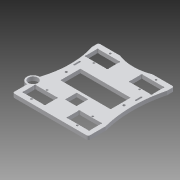
# Autodesk Inventor part: base doble extrusor xl i v1.3
Saved by Autodesk Inventor 2012 SP1 (Build 160190100, 190)
## iProperties
Created: 2015-08-07
Part Number: base doble extrusor xl i v1.3
Material: Default
Document SubType Name: Modeling
Designer: Laser router cnc
Density: 1 g/cm^3
Author: Laser router cnc
Autodesk Inventor part; units mm, degrees
(part 1 of 2)
ref_plane "YZ Plane" through (0, 0, 0) normal (1, 0, 0) x (0, 1, 0)
ref_plane "XZ Plane" through (0, 0, 0) normal (0, 1, 0) x (-1, 0, 0)
ref_plane "XY Plane" through (0, 0, 0) normal (0, 0, 1) x (1, 0, 0)
sketch "Boceto1" plane through (0, 0, 0) normal (0, 0, 1) x (1, 0, 0)
  line L0 (375.8398, -66.6637) -> (375.8398, -81.652)
  line L1 (375.8398, -81.652) -> (361.1315, -81.652)
  line L2 (361.1315, -81.652) -> (361.1315, -66.6637)
  line L3 (361.1315, -66.6637) -> (375.8398, -66.6637)
  line L4 (401.2261, -37.6694) -> (401.2261, -63.2662)
  line L5 (401.2261, -63.2662) -> (336.8198, -63.2662)
  line L6 (336.8198, -63.2662) -> (336.8198, -37.6694)
  line L7 (336.8198, -37.6694) -> (401.2261, -37.6694)
  line L8 (397.7416, -0.2246) -> (397.8694, -0.2311)
  line L9 (397.8694, -0.2311) -> (397.9936, -0.25)
  line L10 (397.9936, -0.25) -> (398.1134, -0.2808)
  line L11 (398.1134, -0.2808) -> (398.2283, -0.3228)
  line L12 (398.2283, -0.3228) -> (398.3376, -0.3754)
  line L13 (398.3376, -0.3754) -> (398.4407, -0.438)
  line L14 (398.4407, -0.438) -> (398.5369, -0.51)
  line L15 (398.5369, -0.51) -> (398.6257, -0.5906)
  line L16 (398.6257, -0.5906) -> (398.7064, -0.6794)
  line L17 (398.7064, -0.6794) -> (398.7784, -0.7756)
  line L18 (398.7784, -0.7756) -> (398.841, -0.8787)
  line L19 (398.841, -0.8787) -> (398.8937, -0.9879)
  line L20 (398.8937, -0.9879) -> (398.9357, -1.1027)
  line L21 (398.9357, -1.1027) -> (398.9665, -1.2225)
  line L22 (398.9665, -1.2225) -> (398.9855, -1.3466)
  line L23 (398.9855, -1.3466) -> (398.9919, -1.4744)
  line L24 (398.9919, -1.4744) -> (398.9855, -1.6022)
  line L25 (398.9855, -1.6022) -> (398.9665, -1.7263)
  line L26 (398.9665, -1.7263) -> (398.9357, -1.8461)
  line L27 (398.9357, -1.8461) -> (398.8937, -1.9609)
  line L28 (398.8937, -1.9609) -> (398.8411, -2.0702)
  line L29 (398.8411, -2.0702) -> (398.7785, -2.1732)
  line L30 (398.7785, -2.1732) -> (398.7065, -2.2695)
  line L31 (398.7065, -2.2695) -> (398.6259, -2.3583)
  line L32 (398.6259, -2.3583) -> (398.5371, -2.4389)
  line L33 (398.5371, -2.4389) -> (398.4409, -2.5109)
  line L34 (398.4409, -2.5109) -> (398.3379, -2.5736)
  line L35 (398.3379, -2.5736) -> (398.2286, -2.6262)
  line L36 (398.2286, -2.6262) -> (398.1138, -2.6683)
  line L37 (398.1138, -2.6683) -> (397.994, -2.6991)
  line L38 (397.994, -2.6991) -> (397.8699, -2.7181)
  line L39 (397.8699, -2.7181) -> (397.7421, -2.7246)
  line L40 (397.7421, -2.7246) -> (397.6143, -2.7182)
  line L41 (397.6143, -2.7182) -> (397.4902, -2.6993)
  line L42 (397.4902, -2.6993) -> (397.3705, -2.6685)
  line L43 (397.3705, -2.6685) -> (397.2556, -2.6265)
  line L44 (397.2556, -2.6265) -> (397.1464, -2.5739)
  line L45 (397.1464, -2.5739) -> (397.0433, -2.5113)
  line L46 (397.0433, -2.5113) -> (396.947, -2.4394)
  line L47 (396.947, -2.4394) -> (396.8583, -2.3587)
  line L48 (396.8583, -2.3587) -> (396.7776, -2.27)
  line L49 (396.7776, -2.27) -> (396.7056, -2.1737)
  line L50 (396.7056, -2.1737) -> (396.643, -2.0707)
  line L51 (396.643, -2.0707) -> (396.5903, -1.9614)
  line L52 (396.5903, -1.9614) -> (396.5482, -1.8466)
  line L53 (396.5482, -1.8466) -> (396.5174, -1.7268)
  line L54 (396.5174, -1.7268) -> (396.4984, -1.6026)
  line L55 (396.4984, -1.6026) -> (396.4919, -1.4748)
  line L56 (396.4919, -1.4748) -> (396.4983, -1.347)
  line L57 (396.4983, -1.347) -> (396.5172, -1.2229)
  line L58 (396.5172, -1.2229) -> (396.548, -1.1031)
  line L59 (396.548, -1.1031) -> (396.59, -0.9883)
  line L60 (396.59, -0.9883) -> (396.6426, -0.879)
  line L61 (396.6426, -0.879) -> (396.7052, -0.776)
  line L62 (396.7052, -0.776) -> (396.7771, -0.6797)
  line L63 (396.7771, -0.6797) -> (396.8578, -0.5909)
  line L64 (396.8578, -0.5909) -> (396.9465, -0.5103)
  line L65 (396.9465, -0.5103) -> (397.0427, -0.4383)
  line L66 (397.0427, -0.4383) -> (397.1458, -0.3756)
  line L67 (397.1458, -0.3756) -> (397.255, -0.323)
  line L68 (397.255, -0.323) -> (397.3699, -0.2809)
  line L69 (397.3699, -0.2809) -> (397.4897, -0.2501)
  line L70 (397.4897, -0.2501) -> (397.6138, -0.2311)
  line L71 (397.6138, -0.2311) -> (397.7416, -0.2246)
  line L72 (397.7416, -21.4052) -> (397.8694, -21.4117)
  line L73 (397.8694, -21.4117) -> (397.9936, -21.4306)
  line L74 (397.9936, -21.4306) -> (398.1134, -21.4614)
  line L75 (398.1134, -21.4614) -> (398.2283, -21.5034)
  line L76 (398.2283, -21.5034) -> (398.3376, -21.5561)
  line L77 (398.3376, -21.5561) -> (398.4407, -21.6187)
  line L78 (398.4407, -21.6187) -> (398.5369, -21.6906)
  line L79 (398.5369, -21.6906) -> (398.6257, -21.7713)
  line L80 (398.6257, -21.7713) -> (398.7064, -21.86)
  line L81 (398.7064, -21.86) -> (398.7784, -21.9562)
  line L82 (398.7784, -21.9562) -> (398.841, -22.0593)
  line L83 (398.841, -22.0593) -> (398.8937, -22.1685)
  line L84 (398.8937, -22.1685) -> (398.9357, -22.2833)
  line L85 (398.9357, -22.2833) -> (398.9665, -22.4031)
  line L86 (398.9665, -22.4031) -> (398.9855, -22.5272)
  line L87 (398.9855, -22.5272) -> (398.9919, -22.655)
  line L88 (398.9919, -22.655) -> (398.9855, -22.7828)
  line L89 (398.9855, -22.7828) -> (398.9665, -22.9069)
  line L90 (398.9665, -22.9069) -> (398.9357, -23.0267)
  line L91 (398.9357, -23.0267) -> (398.8937, -23.1415)
  line L92 (398.8937, -23.1415) -> (398.8411, -23.2508)
  line L93 (398.8411, -23.2508) -> (398.7785, -23.3538)
  line L94 (398.7785, -23.3538) -> (398.7065, -23.4501)
  line L95 (398.7065, -23.4501) -> (398.6259, -23.5389)
  line L96 (398.6259, -23.5389) -> (398.5371, -23.6196)
  line L97 (398.5371, -23.6196) -> (398.4409, -23.6915)
  line L98 (398.4409, -23.6915) -> (398.3379, -23.7542)
  line L99 (398.3379, -23.7542) -> (398.2286, -23.8068)
  line L100 (398.2286, -23.8068) -> (398.1138, -23.8489)
  line L101 (398.1138, -23.8489) -> (397.994, -23.8797)
  line L102 (397.994, -23.8797) -> (397.8699, -23.8987)
  line L103 (397.8699, -23.8987) -> (397.7421, -23.9052)
  line L104 (397.7421, -23.9052) -> (397.6143, -23.8988)
  line L105 (397.6143, -23.8988) -> (397.4902, -23.8799)
  line L106 (397.4902, -23.8799) -> (397.3705, -23.8491)
  line L107 (397.3705, -23.8491) -> (397.2556, -23.8071)
  line L108 (397.2556, -23.8071) -> (397.1464, -23.7545)
  line L109 (397.1464, -23.7545) -> (397.0433, -23.6919)
  line L110 (397.0433, -23.6919) -> (396.947, -23.62)
  line L111 (396.947, -23.62) -> (396.8583, -23.5393)
  line L112 (396.8583, -23.5393) -> (396.7776, -23.4506)
  line L113 (396.7776, -23.4506) -> (396.7056, -23.3544)
  line L114 (396.7056, -23.3544) -> (396.643, -23.2513)
  line L115 (396.643, -23.2513) -> (396.5903, -23.142)
  line L116 (396.5903, -23.142) -> (396.5482, -23.0272)
  line L117 (396.5482, -23.0272) -> (396.5174, -22.9074)
  line L118 (396.5174, -22.9074) -> (396.4984, -22.7833)
  line L119 (396.4984, -22.7833) -> (396.4919, -22.6554)
  line L120 (396.4919, -22.6554) -> (396.4983, -22.5276)
  line L121 (396.4983, -22.5276) -> (396.5172, -22.4035)
  line L122 (396.5172, -22.4035) -> (396.548, -22.2838)
  line L123 (396.548, -22.2838) -> (396.59, -22.1689)
  line L124 (396.59, -22.1689) -> (396.6426, -22.0596)
  line L125 (396.6426, -22.0596) -> (396.7052, -21.9566)
  line L126 (396.7052, -21.9566) -> (396.7771, -21.8603)
  line L127 (396.7771, -21.8603) -> (396.8578, -21.7716)
  line L128 (396.8578, -21.7716) -> (396.9465, -21.6909)
  line L129 (396.9465, -21.6909) -> (397.0427, -21.6189)
  line L130 (397.0427, -21.6189) -> (397.1458, -21.5563)
  line L131 (397.1458, -21.5563) -> (397.255, -21.5036)
  line L132 (397.255, -21.5036) -> (397.3699, -21.4615)
  line L133 (397.3699, -21.4615) -> (397.4897, -21.4307)
  line L134 (397.4897, -21.4307) -> (397.6138, -21.4117)
  line L135 (397.6138, -21.4117) -> (397.7416, -21.4052)
  line L136 (329.5431, -30.1414) -> (329.5379, -30.0405)
  line L137 (329.5379, -30.0405) -> (329.5228, -29.9424)
  line L138 (329.5228, -29.9424) -> (329.4981, -29.8475)
  line L139 (329.4981, -29.8475) -> (329.4644, -29.7565)
  line L140 (329.4644, -29.7565) -> (329.4223, -29.6699)
  line L141 (329.4223, -29.6699) -> (329.3722, -29.5881)
  line L142 (329.3722, -29.5881) -> (329.3146, -29.5116)
  line L143 (329.3146, -29.5116) -> (329.25, -29.441)
  line L144 (329.25, -29.441) -> (329.179, -29.3768)
  line L145 (329.179, -29.3768) -> (329.102, -29.3195)
  line L146 (329.102, -29.3195) -> (329.0195, -29.2695)
  line L147 (329.0195, -29.2695) -> (328.9321, -29.2276)
  line L148 (328.9321, -29.2276) -> (328.8402, -29.194)
  line L149 (328.8402, -29.194) -> (328.7443, -29.1694)
  line L150 (328.7443, -29.1694) -> (328.645, -29.1543)
  line L151 (328.645, -29.1543) -> (328.5427, -29.1491)
  line L152 (328.5427, -29.1491) -> (328.4404, -29.1543)
  line L153 (328.4404, -29.1543) -> (328.3411, -29.1694)
  line L154 (328.3411, -29.1694) -> (328.2453, -29.194)
  line L155 (328.2453, -29.194) -> (328.1534, -29.2276)
  line L156 (328.1534, -29.2276) -> (328.066, -29.2696)
  line L157 (328.066, -29.2696) -> (327.9835, -29.3196)
  line L158 (327.9835, -29.3196) -> (327.9065, -29.3769)
  line L159 (327.9065, -29.3769) -> (327.8355, -29.4411)
  line L160 (327.8355, -29.4411) -> (327.7709, -29.5118)
  line L161 (327.7709, -29.5118) -> (327.7134, -29.5883)
  line L162 (327.7134, -29.5883) -> (327.6633, -29.6701)
  line L163 (327.6633, -29.6701) -> (327.6212, -29.7568)
  line L164 (327.6212, -29.7568) -> (327.5875, -29.8478)
  line L165 (327.5875, -29.8478) -> (327.5629, -29.9426)
  line L166 (327.5629, -29.9426) -> (327.5477, -30.0407)
  line L167 (327.5477, -30.0407) -> (327.5426, -30.1416)
  line L168 (327.5426, -30.1416) -> (327.5426, -37.1435)
  line L169 (327.5426, -37.1435) -> (327.5478, -37.2444)
  line L170 (327.5478, -37.2444) -> (327.5629, -37.3425)
  line L171 (327.5629, -37.3425) -> (327.5876, -37.4373)
  line L172 (327.5876, -37.4373) -> (327.6213, -37.5283)
  line L173 (327.6213, -37.5283) -> (327.6634, -37.615)
  line L174 (327.6634, -37.615) -> (327.7135, -37.6968)
  line L175 (327.7135, -37.6968) -> (327.7711, -37.7733)
  line L176 (327.7711, -37.7733) -> (327.8357, -37.8439)
  line L177 (327.8357, -37.8439) -> (327.9067, -37.9081)
  line L178 (327.9067, -37.9081) -> (327.9837, -37.9654)
  line L179 (327.9837, -37.9654) -> (328.0662, -38.0153)
  line L180 (328.0662, -38.0153) -> (328.1536, -38.0573)
  line L181 (328.1536, -38.0573) -> (328.2455, -38.0909)
  line L182 (328.2455, -38.0909) -> (328.3414, -38.1155)
  line L183 (328.3414, -38.1155) -> (328.4407, -38.1306)
  line L184 (328.4407, -38.1306) -> (328.543, -38.1358)
  line L185 (328.543, -38.1358) -> (328.6453, -38.1306)
  line L186 (328.6453, -38.1306) -> (328.7446, -38.1155)
  line L187 (328.7446, -38.1155) -> (328.8404, -38.0909)
  line L188 (328.8404, -38.0909) -> (328.9323, -38.0573)
  line L189 (328.9323, -38.0573) -> (329.0197, -38.0153)
  line L190 (329.0197, -38.0153) -> (329.1022, -37.9654)
  line L191 (329.1022, -37.9654) -> (329.1792, -37.908)
  line L192 (329.1792, -37.908) -> (329.2502, -37.8438)
  line L193 (329.2502, -37.8438) -> (329.3148, -37.7732)
  line L194 (329.3148, -37.7732) -> (329.3723, -37.6967)
  line L195 (329.3723, -37.6967) -> (329.4224, -37.6148)
  line L196 (329.4224, -37.6148) -> (329.4645, -37.5281)
  line L197 (329.4645, -37.5281) -> (329.4982, -37.4371)
  line L198 (329.4982, -37.4371) -> (329.5228, -37.3423)
  line L199 (329.5228, -37.3423) -> (329.538, -37.2442)
  line L200 (329.538, -37.2442) -> (329.5431, -37.1434)
  line L201 (329.5431, -37.1434) -> (329.5431, -30.1414)
  line L202 (408.58, -30.1812) -> (408.5747, -30.0814)
  line L203 (408.5747, -30.0814) -> (408.5592, -29.9844)
  line L204 (408.5592, -29.9844) -> (408.5339, -29.8907)
  line L205 (408.5339, -29.8907) -> (408.4994, -29.8007)
  line L206 (408.4994, -29.8007) -> (408.4562, -29.715)
  line L207 (408.4562, -29.715) -> (408.4049, -29.6341)
  line L208 (408.4049, -29.6341) -> (408.3459, -29.5585)
  line L209 (408.3459, -29.5585) -> (408.2797, -29.4887)
  line L210 (408.2797, -29.4887) -> (408.2069, -29.4252)
  line L211 (408.2069, -29.4252) -> (408.128, -29.3685)
  line L212 (408.128, -29.3685) -> (408.0435, -29.3192)
  line L213 (408.0435, -29.3192) -> (407.9539, -29.2776)
  line L214 (407.9539, -29.2776) -> (407.8597, -29.2445)
  line L215 (407.8597, -29.2445) -> (407.7615, -29.2201)
  line L216 (407.7615, -29.2201) -> (407.6597, -29.2052)
  line L217 (407.6597, -29.2052) -> (407.5549, -29.2001)
  line L218 (407.5549, -29.2001) -> (407.4501, -29.2052)
  line L219 (407.4501, -29.2052) -> (407.3484, -29.2202)
  line L220 (407.3484, -29.2202) -> (407.2501, -29.2445)
  line L221 (407.2501, -29.2445) -> (407.156, -29.2777)
  line L222 (407.156, -29.2777) -> (407.0664, -29.3192)
  line L223 (407.0664, -29.3192) -> (406.9819, -29.3686)
  line L224 (406.9819, -29.3686) -> (406.903, -29.4253)
  line L225 (406.903, -29.4253) -> (406.8302, -29.4888)
  line L226 (406.8302, -29.4888) -> (406.7641, -29.5587)
  line L227 (406.7641, -29.5587) -> (406.7051, -29.6343)
  line L228 (406.7051, -29.6343) -> (406.6538, -29.7152)
  line L229 (406.6538, -29.7152) -> (406.6106, -29.8009)
  line L230 (406.6106, -29.8009) -> (406.5762, -29.8909)
  line L231 (406.5762, -29.8909) -> (406.5509, -29.9846)
  line L232 (406.5509, -29.9846) -> (406.5354, -30.0816)
  line L233 (406.5354, -30.0816) -> (406.5301, -30.1814)
  line L234 (406.5301, -30.1814) -> (406.5322, -37.1078)
  line L235 (406.5322, -37.1078) -> (406.5301, -37.2452)
  line L236 (406.5301, -37.2452) -> (406.5477, -37.38)
  line L237 (406.5477, -37.38) -> (406.584, -37.5104)
  line L238 (406.584, -37.5104) -> (406.6383, -37.6345)
  line L239 (406.6383, -37.6345) -> (406.7096, -37.7506)
  line L240 (406.7096, -37.7506) -> (406.7969, -37.8568)
  line L241 (406.7969, -37.8568) -> (406.8996, -37.9514)
  line L242 (406.8996, -37.9514) -> (407.0166, -38.0325)
  line L243 (407.0166, -38.0325) -> (407.1441, -38.0971)
  line L244 (407.1441, -38.0971) -> (407.2777, -38.1432)
  line L245 (407.2777, -38.1432) -> (407.4154, -38.1709)
  line L246 (407.4154, -38.1709) -> (407.5552, -38.1801)
  line L247 (407.5552, -38.1801) -> (407.6949, -38.1708)
  line L248 (407.6949, -38.1708) -> (407.8326, -38.1431)
  line L249 (407.8326, -38.1431) -> (407.9663, -38.097)
  line L250 (407.9663, -38.097) -> (408.0938, -38.0324)
  line L251 (408.0938, -38.0324) -> (408.2107, -37.9512)
  line L252 (408.2107, -37.9512) -> (408.3133, -37.8566)
  line L253 (408.3133, -37.8566) -> (408.4007, -37.7504)
  line L254 (408.4007, -37.7504) -> (408.472, -37.6342)
  line L255 (408.472, -37.6342) -> (408.5262, -37.5101)
  line L256 (408.5262, -37.5101) -> (408.5625, -37.3798)
  line L257 (408.5625, -37.3798) -> (408.5801, -37.245)
  line L258 (408.5801, -37.245) -> (408.578, -37.1077)
  line L259 (408.578, -37.1077) -> (408.58, -30.1812)
  line L260 (339.1203, -21.4052) -> (339.2481, -21.4117)
  line L261 (339.2481, -21.4117) -> (339.3723, -21.4306)
  line L262 (339.3723, -21.4306) -> (339.4921, -21.4614)
  line L263 (339.4921, -21.4614) -> (339.607, -21.5034)
  line L264 (339.607, -21.5034) -> (339.7163, -21.5561)
  line L265 (339.7163, -21.5561) -> (339.8194, -21.6187)
  line L266 (339.8194, -21.6187) -> (339.9156, -21.6906)
  line L267 (339.9156, -21.6906) -> (340.0044, -21.7713)
  line L268 (340.0044, -21.7713) -> (340.0851, -21.86)
  line L269 (340.0851, -21.86) -> (340.1571, -21.9562)
  line L270 (340.1571, -21.9562) -> (340.2197, -22.0593)
  line L271 (340.2197, -22.0593) -> (340.2723, -22.1685)
  line L272 (340.2723, -22.1685) -> (340.3144, -22.2833)
  line L273 (340.3144, -22.2833) -> (340.3452, -22.4031)
  line L274 (340.3452, -22.4031) -> (340.3641, -22.5272)
  line L275 (340.3641, -22.5272) -> (340.3706, -22.655)
  line L276 (340.3706, -22.655) -> (340.3641, -22.7828)
  line L277 (340.3641, -22.7828) -> (340.3452, -22.9069)
  line L278 (340.3452, -22.9069) -> (340.3144, -23.0267)
  line L279 (340.3144, -23.0267) -> (340.2724, -23.1415)
  line L280 (340.2724, -23.1415) -> (340.2198, -23.2508)
  line L281 (340.2198, -23.2508) -> (340.1572, -23.3538)
  line L282 (340.1572, -23.3538) -> (340.0852, -23.4501)
  line L283 (340.0852, -23.4501) -> (340.0046, -23.5389)
  line L284 (340.0046, -23.5389) -> (339.9158, -23.6196)
  line L285 (339.9158, -23.6196) -> (339.8196, -23.6915)
  line L286 (339.8196, -23.6915) -> (339.7165, -23.7542)
  line L287 (339.7165, -23.7542) -> (339.6073, -23.8068)
  line L288 (339.6073, -23.8068) -> (339.4925, -23.8489)
  line L289 (339.4925, -23.8489) -> (339.3727, -23.8797)
  line L290 (339.3727, -23.8797) -> (339.2486, -23.8987)
  line L291 (339.2486, -23.8987) -> (339.1208, -23.9052)
  line L292 (339.1208, -23.9052) -> (338.993, -23.8988)
  line L293 (338.993, -23.8988) -> (338.8689, -23.8799)
  line L294 (338.8689, -23.8799) -> (338.7491, -23.8491)
  line L295 (338.7491, -23.8491) -> (338.6343, -23.8071)
  line L296 (338.6343, -23.8071) -> (338.525, -23.7545)
  line L297 (338.525, -23.7545) -> (338.422, -23.6919)
  line L298 (338.422, -23.6919) -> (338.3257, -23.62)
  line L299 (338.3257, -23.62) -> (338.2369, -23.5393)
  line L300 (338.2369, -23.5393) -> (338.1563, -23.4506)
  line L301 (338.1563, -23.4506) -> (338.0843, -23.3544)
  line L302 (338.0843, -23.3544) -> (338.0216, -23.2513)
  line L303 (338.0216, -23.2513) -> (337.969, -23.142)
  line L304 (337.969, -23.142) -> (337.9269, -23.0272)
  line L305 (337.9269, -23.0272) -> (337.8961, -22.9074)
  line L306 (337.8961, -22.9074) -> (337.8771, -22.7833)
  line L307 (337.8771, -22.7833) -> (337.8706, -22.6554)
  line L308 (337.8706, -22.6554) -> (337.877, -22.5276)
  line L309 (337.877, -22.5276) -> (337.8959, -22.4035)
  line L310 (337.8959, -22.4035) -> (337.9267, -22.2838)
  line L311 (337.9267, -22.2838) -> (337.9687, -22.1689)
  line L312 (337.9687, -22.1689) -> (338.0213, -22.0596)
  line L313 (338.0213, -22.0596) -> (338.0839, -21.9566)
  line L314 (338.0839, -21.9566) -> (338.1558, -21.8603)
  line L315 (338.1558, -21.8603) -> (338.2365, -21.7716)
  line L316 (338.2365, -21.7716) -> (338.3252, -21.6909)
  line L317 (338.3252, -21.6909) -> (338.4214, -21.6189)
  line L318 (338.4214, -21.6189) -> (338.5245, -21.5563)
  line L319 (338.5245, -21.5563) -> (338.6337, -21.5036)
  line L320 (338.6337, -21.5036) -> (338.7486, -21.4615)
  line L321 (338.7486, -21.4615) -> (338.8684, -21.4307)
  line L322 (338.8684, -21.4307) -> (338.9925, -21.4117)
  line L323 (338.9925, -21.4117) -> (339.1203, -21.4052)
  line L324 (339.1203, -0.3834) -> (339.2481, -0.3898)
  line L325 (339.2481, -0.3898) -> (339.3723, -0.4088)
  line L326 (339.3723, -0.4088) -> (339.4921, -0.4396)
  line L327 (339.4921, -0.4396) -> (339.607, -0.4816)
  line L328 (339.607, -0.4816) -> (339.7163, -0.5342)
  line L329 (339.7163, -0.5342) -> (339.8194, -0.5968)
  line L330 (339.8194, -0.5968) -> (339.9156, -0.6688)
  line L331 (339.9156, -0.6688) -> (340.0044, -0.7494)
  line L332 (340.0044, -0.7494) -> (340.0851, -0.8382)
  line L333 (340.0851, -0.8382) -> (340.1571, -0.9344)
  line L334 (340.1571, -0.9344) -> (340.2197, -1.0374)
  line L335 (340.2197, -1.0374) -> (340.2723, -1.1467)
  line L336 (340.2723, -1.1467) -> (340.3144, -1.2615)
  line L337 (340.3144, -1.2615) -> (340.3452, -1.3813)
  line L338 (340.3452, -1.3813) -> (340.3641, -1.5054)
  line L339 (340.3641, -1.5054) -> (340.3706, -1.6332)
  line L340 (340.3706, -1.6332) -> (340.3641, -1.7609)
  line L341 (340.3641, -1.7609) -> (340.3452, -1.885)
  line L342 (340.3452, -1.885) -> (340.3144, -2.0048)
  line L343 (340.3144, -2.0048) -> (340.2724, -2.1197)
  line L344 (340.2724, -2.1197) -> (340.2198, -2.2289)
  line L345 (340.2198, -2.2289) -> (340.1572, -2.332)
  line L346 (340.1572, -2.332) -> (340.0852, -2.4282)
  line L347 (340.0852, -2.4282) -> (340.0046, -2.517)
  line L348 (340.0046, -2.517) -> (339.9158, -2.5977)
  line L349 (339.9158, -2.5977) -> (339.8196, -2.6697)
  line L350 (339.8196, -2.6697) -> (339.7165, -2.7323)
  line L351 (339.7165, -2.7323) -> (339.6073, -2.785)
  line L352 (339.6073, -2.785) -> (339.4925, -2.8271)
  line L353 (339.4925, -2.8271) -> (339.3727, -2.8579)
  line L354 (339.3727, -2.8579) -> (339.2486, -2.8769)
  line L355 (339.2486, -2.8769) -> (339.1208, -2.8834)
  line L356 (339.1208, -2.8834) -> (338.993, -2.877)
  line L357 (338.993, -2.877) -> (338.8689, -2.8581)
  line L358 (338.8689, -2.8581) -> (338.7491, -2.8273)
  line L359 (338.7491, -2.8273) -> (338.6343, -2.7853)
  line L360 (338.6343, -2.7853) -> (338.525, -2.7327)
  line L361 (338.525, -2.7327) -> (338.422, -2.6701)
  line L362 (338.422, -2.6701) -> (338.3257, -2.5982)
  line L363 (338.3257, -2.5982) -> (338.2369, -2.5175)
  line L364 (338.2369, -2.5175) -> (338.1563, -2.4287)
  line L365 (338.1563, -2.4287) -> (338.0843, -2.3325)
  line L366 (338.0843, -2.3325) -> (338.0216, -2.2295)
  line L367 (338.0216, -2.2295) -> (337.969, -2.1202)
  line L368 (337.969, -2.1202) -> (337.9269, -2.0053)
  line L369 (337.9269, -2.0053) -> (337.8961, -1.8855)
  line L370 (337.8961, -1.8855) -> (337.8771, -1.7614)
  line L371 (337.8771, -1.7614) -> (337.8706, -1.6336)
  line L372 (337.8706, -1.6336) -> (337.877, -1.5058)
  line L373 (337.877, -1.5058) -> (337.8959, -1.3817)
  line L374 (337.8959, -1.3817) -> (337.9267, -1.2619)
  line L375 (337.9267, -1.2619) -> (337.9687, -1.1471)
  line L376 (337.9687, -1.1471) -> (338.0213, -1.0378)
  line L377 (338.0213, -1.0378) -> (338.0839, -0.9347)
  line L378 (338.0839, -0.9347) -> (338.1558, -0.8385)
  line L379 (338.1558, -0.8385) -> (338.2365, -0.7497)
  line L380 (338.2365, -0.7497) -> (338.3252, -0.669)
  line L381 (338.3252, -0.669) -> (338.4214, -0.597)
  line L382 (338.4214, -0.597) -> (338.5245, -0.5344)
  line L383 (338.5245, -0.5344) -> (338.6337, -0.4817)
  line L384 (338.6337, -0.4817) -> (338.7486, -0.4397)
  line L385 (338.7486, -0.4397) -> (338.8684, -0.4088)
  line L386 (338.8684, -0.4088) -> (338.9925, -0.3899)
  line L387 (338.9925, -0.3899) -> (339.1203, -0.3834)
  line L388 (397.7416, -81.3905) -> (397.8694, -81.3969)
  line L389 (397.8694, -81.3969) -> (397.9936, -81.4159)
  line L390 (397.9936, -81.4159) -> (398.1134, -81.4467)
  line L391 (398.1134, -81.4467) -> (398.2283, -81.4887)
  line L392 (398.2283, -81.4887) -> (398.3376, -81.5413)
  line L393 (398.3376, -81.5413) -> (398.4407, -81.6039)
  line L394 (398.4407, -81.6039) -> (398.5369, -81.6759)
  line L395 (398.5369, -81.6759) -> (398.6257, -81.7565)
  line L396 (398.6257, -81.7565) -> (398.7064, -81.8453)
  line L397 (398.7064, -81.8453) -> (398.7784, -81.9415)
  line L398 (398.7784, -81.9415) -> (398.841, -82.0445)
  line L399 (398.841, -82.0445) -> (398.8937, -82.1538)
  line L400 (398.8937, -82.1538) -> (398.9357, -82.2686)
  line L401 (398.9357, -82.2686) -> (398.9665, -82.3884)
  line L402 (398.9665, -82.3884) -> (398.9855, -82.5125)
  line L403 (398.9855, -82.5125) -> (398.9919, -82.6403)
  line L404 (398.9919, -82.6403) -> (398.9855, -82.7681)
  line L405 (398.9855, -82.7681) -> (398.9665, -82.8922)
  line L406 (398.9665, -82.8922) -> (398.9357, -83.0119)
  line L407 (398.9357, -83.0119) -> (398.8937, -83.1268)
  line L408 (398.8937, -83.1268) -> (398.8411, -83.2361)
  line L409 (398.8411, -83.2361) -> (398.7785, -83.3391)
  line L410 (398.7785, -83.3391) -> (398.7065, -83.4354)
  line L411 (398.7065, -83.4354) -> (398.6259, -83.5241)
  line L412 (398.6259, -83.5241) -> (398.5371, -83.6048)
  line L413 (398.5371, -83.6048) -> (398.4409, -83.6768)
  line L414 (398.4409, -83.6768) -> (398.3379, -83.7395)
  line L415 (398.3379, -83.7395) -> (398.2286, -83.7921)
  line L416 (398.2286, -83.7921) -> (398.1138, -83.8342)
  line L417 (398.1138, -83.8342) -> (397.994, -83.865)
  line L418 (397.994, -83.865) -> (397.8699, -83.884)
  line L419 (397.8699, -83.884) -> (397.7421, -83.8905)
  line L420 (397.7421, -83.8905) -> (397.6143, -83.8841)
  line L421 (397.6143, -83.8841) -> (397.4902, -83.8652)
  line L422 (397.4902, -83.8652) -> (397.3705, -83.8344)
  line L423 (397.3705, -83.8344) -> (397.2556, -83.7924)
  line L424 (397.2556, -83.7924) -> (397.1464, -83.7398)
  line L425 (397.1464, -83.7398) -> (397.0433, -83.6772)
  line L426 (397.0433, -83.6772) -> (396.947, -83.6053)
  line L427 (396.947, -83.6053) -> (396.8583, -83.5246)
  line L428 (396.8583, -83.5246) -> (396.7776, -83.4359)
  line L429 (396.7776, -83.4359) -> (396.7056, -83.3396)
  line L430 (396.7056, -83.3396) -> (396.643, -83.2366)
  line L431 (396.643, -83.2366) -> (396.5903, -83.1273)
  line L432 (396.5903, -83.1273) -> (396.5482, -83.0125)
  line L433 (396.5482, -83.0125) -> (396.5174, -82.8927)
  line L434 (396.5174, -82.8927) -> (396.4984, -82.7685)
  line L435 (396.4984, -82.7685) -> (396.4919, -82.6407)
  line L436 (396.4919, -82.6407) -> (396.4983, -82.5129)
  line L437 (396.4983, -82.5129) -> (396.5172, -82.3888)
  line L438 (396.5172, -82.3888) -> (396.548, -82.269)
  line L439 (396.548, -82.269) -> (396.59, -82.1542)
  line L440 (396.59, -82.1542) -> (396.6426, -82.0449)
  line L441 (396.6426, -82.0449) -> (396.7052, -81.9419)
  line L442 (396.7052, -81.9419) -> (396.7771, -81.8456)
  line L443 (396.7771, -81.8456) -> (396.8578, -81.7568)
  line L444 (396.8578, -81.7568) -> (396.9465, -81.6761)
  line L445 (396.9465, -81.6761) -> (397.0427, -81.6042)
  line L446 (397.0427, -81.6042) -> (397.1458, -81.5415)
  line L447 (397.1458, -81.5415) -> (397.255, -81.4889)
  line L448 (397.255, -81.4889) -> (397.3699, -81.4468)
  line L449 (397.3699, -81.4468) -> (397.4897, -81.416)
  line L450 (397.4897, -81.416) -> (397.6138, -81.397)
  line L451 (397.6138, -81.397) -> (397.7416, -81.3905)
  line L452 (339.1203, -81.3905) -> (339.2481, -81.3969)
  line L453 (339.2481, -81.3969) -> (339.3723, -81.4159)
  line L454 (339.3723, -81.4159) -> (339.4921, -81.4467)
  line L455 (339.4921, -81.4467) -> (339.607, -81.4887)
  line L456 (339.607, -81.4887) -> (339.7163, -81.5413)
  line L457 (339.7163, -81.5413) -> (339.8194, -81.6039)
  line L458 (339.8194, -81.6039) -> (339.9156, -81.6759)
  line L459 (339.9156, -81.6759) -> (340.0044, -81.7565)
  line L460 (340.0044, -81.7565) -> (340.0851, -81.8453)
  line L461 (340.0851, -81.8453) -> (340.1571, -81.9415)
  line L462 (340.1571, -81.9415) -> (340.2197, -82.0445)
  line L463 (340.2197, -82.0445) -> (340.2723, -82.1538)
  line L464 (340.2723, -82.1538) -> (340.3144, -82.2686)
  line L465 (340.3144, -82.2686) -> (340.3452, -82.3884)
  line L466 (340.3452, -82.3884) -> (340.3641, -82.5125)
  line L467 (340.3641, -82.5125) -> (340.3706, -82.6403)
  line L468 (340.3706, -82.6403) -> (340.3641, -82.7681)
  line L469 (340.3641, -82.7681) -> (340.3452, -82.8922)
  line L470 (340.3452, -82.8922) -> (340.3144, -83.0119)
  line L471 (340.3144, -83.0119) -> (340.2724, -83.1268)
  line L472 (340.2724, -83.1268) -> (340.2198, -83.2361)
  line L473 (340.2198, -83.2361) -> (340.1572, -83.3391)
  line L474 (340.1572, -83.3391) -> (340.0852, -83.4354)
  line L475 (340.0852, -83.4354) -> (340.0046, -83.5241)
  line L476 (340.0046, -83.5241) -> (339.9158, -83.6048)
  line L477 (339.9158, -83.6048) -> (339.8196, -83.6768)
  line L478 (339.8196, -83.6768) -> (339.7165, -83.7395)
  line L479 (339.7165, -83.7395) -> (339.6073, -83.7921)
  line L480 (339.6073, -83.7921) -> (339.4925, -83.8342)
  line L481 (339.4925, -83.8342) -> (339.3727, -83.865)
  line L482 (339.3727, -83.865) -> (339.2486, -83.884)
  line L483 (339.2486, -83.884) -> (339.1208, -83.8905)
  line L484 (339.1208, -83.8905) -> (338.993, -83.8841)
  line L485 (338.993, -83.8841) -> (338.8689, -83.8652)
  line L486 (338.8689, -83.8652) -> (338.7491, -83.8344)
  line L487 (338.7491, -83.8344) -> (338.6343, -83.7924)
  line L488 (338.6343, -83.7924) -> (338.525, -83.7398)
  line L489 (338.525, -83.7398) -> (338.422, -83.6772)
  line L490 (338.422, -83.6772) -> (338.3257, -83.6053)
  line L491 (338.3257, -83.6053) -> (338.2369, -83.5246)
  line L492 (338.2369, -83.5246) -> (338.1563, -83.4359)
  line L493 (338.1563, -83.4359) -> (338.0843, -83.3396)
  line L494 (338.0843, -83.3396) -> (338.0216, -83.2366)
  line L495 (338.0216, -83.2366) -> (337.969, -83.1273)
  line L496 (337.969, -83.1273) -> (337.9269, -83.0125)
  line L497 (337.9269, -83.0125) -> (337.8961, -82.8927)
  line L498 (337.8961, -82.8927) -> (337.8771, -82.7685)
  line L499 (337.8771, -82.7685) -> (337.8706, -82.6407)
  line L500 (337.8706, -82.6407) -> (337.877, -82.5129)
  line L501 (337.877, -82.5129) -> (337.8959, -82.3888)
  line L502 (337.8959, -82.3888) -> (337.9267, -82.269)
  line L503 (337.9267, -82.269) -> (337.9687, -82.1542)
  line L504 (337.9687, -82.1542) -> (338.0213, -82.0449)
  line L505 (338.0213, -82.0449) -> (338.0839, -81.9419)
  line L506 (338.0839, -81.9419) -> (338.1558, -81.8456)
  line L507 (338.1558, -81.8456) -> (338.2365, -81.7568)
  line L508 (338.2365, -81.7568) -> (338.3252, -81.6761)
  line L509 (338.3252, -81.6761) -> (338.4214, -81.6042)
  line L510 (338.4214, -81.6042) -> (338.5245, -81.5415)
  line L511 (338.5245, -81.5415) -> (338.6337, -81.4889)
  line L512 (338.6337, -81.4889) -> (338.7486, -81.4468)
  line L513 (338.7486, -81.4468) -> (338.8684, -81.416)
  line L514 (338.8684, -81.416) -> (338.9925, -81.397)
  line L515 (338.9925, -81.397) -> (339.1203, -81.3905)
  line L516 (339.1203, -101.3962) -> (339.2481, -101.4026)
  line L517 (339.2481, -101.4026) -> (339.3722, -101.4216)
  line L518 (339.3722, -101.4216) -> (339.4921, -101.4523)
  line L519 (339.4921, -101.4523) -> (339.6069, -101.4944)
  line L520 (339.6069, -101.4944) -> (339.7162, -101.547)
  line L521 (339.7162, -101.547) -> (339.8193, -101.6096)
  line L522 (339.8193, -101.6096) -> (339.9156, -101.6815)
  line L523 (339.9156, -101.6815) -> (340.0044, -101.7622)
  line L524 (340.0044, -101.7622) -> (340.0851, -101.8509)
  line L525 (340.0851, -101.8509) -> (340.1571, -101.9471)
  line L526 (340.1571, -101.9471) -> (340.2197, -102.0502)
  line L527 (340.2197, -102.0502) -> (340.2723, -102.1594)
  line L528 (340.2723, -102.1594) -> (340.3144, -102.2743)
  line L529 (340.3144, -102.2743) -> (340.3452, -102.394)
  line L530 (340.3452, -102.394) -> (340.3641, -102.5181)
  line L531 (340.3641, -102.5181) -> (340.3706, -102.646)
  line L532 (340.3706, -102.646) -> (340.3641, -102.7738)
  line L533 (340.3641, -102.7738) -> (340.3452, -102.8979)
  line L534 (340.3452, -102.8979) -> (340.3144, -103.0177)
  line L535 (340.3144, -103.0177) -> (340.2724, -103.1325)
  line L536 (340.2724, -103.1325) -> (340.2198, -103.2418)
  line L537 (340.2198, -103.2418) -> (340.1572, -103.3449)
  line L538 (340.1572, -103.3449) -> (340.0853, -103.4411)
  line L539 (340.0853, -103.4411) -> (340.0046, -103.5299)
  line L540 (340.0046, -103.5299) -> (339.9159, -103.6106)
  line L541 (339.9159, -103.6106) -> (339.8196, -103.6825)
  line L542 (339.8196, -103.6825) -> (339.7166, -103.7452)
  line L543 (339.7166, -103.7452) -> (339.6073, -103.7978)
  line L544 (339.6073, -103.7978) -> (339.4925, -103.8399)
  line L545 (339.4925, -103.8399) -> (339.3727, -103.8707)
  line L546 (339.3727, -103.8707) -> (339.2486, -103.8897)
  line L547 (339.2486, -103.8897) -> (339.1208, -103.8962)
  line L548 (339.1208, -103.8962) -> (338.993, -103.8898)
  line L549 (338.993, -103.8898) -> (338.8689, -103.8708)
  line L550 (338.8689, -103.8708) -> (338.7491, -103.8401)
  line L551 (338.7491, -103.8401) -> (338.6342, -103.7981)
  line L552 (338.6342, -103.7981) -> (338.525, -103.7454)
  line L553 (338.525, -103.7454) -> (338.4219, -103.6829)
  line L554 (338.4219, -103.6829) -> (338.3257, -103.6109)
  line L555 (338.3257, -103.6109) -> (338.2369, -103.5302)
  line L556 (338.2369, -103.5302) -> (338.1562, -103.4415)
  line L557 (338.1562, -103.4415) -> (338.0842, -103.3453)
  line L558 (338.0842, -103.3453) -> (338.0216, -103.2422)
  line L559 (338.0216, -103.2422) -> (337.9689, -103.1329)
  line L560 (337.9689, -103.1329) -> (337.9269, -103.0181)
  line L561 (337.9269, -103.0181) -> (337.8961, -102.8983)
  line L562 (337.8961, -102.8983) -> (337.8771, -102.7742)
  line L563 (337.8771, -102.7742) -> (337.8706, -102.6464)
  line L564 (337.8706, -102.6464) -> (337.877, -102.5186)
  line L565 (337.877, -102.5186) -> (337.8959, -102.3945)
  line L566 (337.8959, -102.3945) -> (337.9267, -102.2747)
  line L567 (337.9267, -102.2747) -> (337.9687, -102.1599)
  line L568 (337.9687, -102.1599) -> (338.0213, -102.0506)
  line L569 (338.0213, -102.0506) -> (338.0838, -101.9476)
  line L570 (338.0838, -101.9476) -> (338.1558, -101.8513)
  line L571 (338.1558, -101.8513) -> (338.2364, -101.7625)
  line L572 (338.2364, -101.7625) -> (338.3252, -101.6818)
  line L573 (338.3252, -101.6818) -> (338.4214, -101.6099)
  line L574 (338.4214, -101.6099) -> (338.5244, -101.5472)
  line L575 (338.5244, -101.5472) -> (338.6337, -101.4945)
  line L576 (338.6337, -101.4945) -> (338.7485, -101.4525)
  line L577 (338.7485, -101.4525) -> (338.8683, -101.4216)
  line L578 (338.8683, -101.4216) -> (338.9925, -101.4027)
  line L579 (338.9925, -101.4027) -> (339.1203, -101.3962)
  line L580 (397.7416, -101.3962) -> (397.8694, -101.4026)
  line L581 (397.8694, -101.4026) -> (397.9936, -101.4216)
  line L582 (397.9936, -101.4216) -> (398.1134, -101.4524)
  line L583 (398.1134, -101.4524) -> (398.2283, -101.4944)
  line L584 (398.2283, -101.4944) -> (398.3376, -101.547)
  line L585 (398.3376, -101.547) -> (398.4407, -101.6096)
  line L586 (398.4407, -101.6096) -> (398.5369, -101.6815)
  line L587 (398.5369, -101.6815) -> (398.6257, -101.7622)
  line L588 (398.6257, -101.7622) -> (398.7064, -101.851)
  line L589 (398.7064, -101.851) -> (398.7784, -101.9472)
  line L590 (398.7784, -101.9472) -> (398.841, -102.0502)
  line L591 (398.841, -102.0502) -> (398.8937, -102.1595)
  line L592 (398.8937, -102.1595) -> (398.9357, -102.2743)
  line L593 (398.9357, -102.2743) -> (398.9665, -102.3941)
  line L594 (398.9665, -102.3941) -> (398.9855, -102.5182)
  line L595 (398.9855, -102.5182) -> (398.9919, -102.6459)
  line L596 (398.9919, -102.6459) -> (398.9855, -102.7737)
  line L597 (398.9855, -102.7737) -> (398.9665, -102.8978)
  line L598 (398.9665, -102.8978) -> (398.9357, -103.0176)
  line L599 (398.9357, -103.0176) -> (398.8937, -103.1325)
  line L600 (398.8937, -103.1325) -> (398.8411, -103.2417)
  line L601 (398.8411, -103.2417) -> (398.7785, -103.3448)
  line L602 (398.7785, -103.3448) -> (398.7065, -103.441)
  line L603 (398.7065, -103.441) -> (398.6259, -103.5298)
  line L604 (398.6259, -103.5298) -> (398.5371, -103.6105)
  line L605 (398.5371, -103.6105) -> (398.4409, -103.6825)
  line L606 (398.4409, -103.6825) -> (398.3379, -103.7451)
  line L607 (398.3379, -103.7451) -> (398.2286, -103.7978)
  line L608 (398.2286, -103.7978) -> (398.1138, -103.8399)
  line L609 (398.1138, -103.8399) -> (397.994, -103.8707)
  line L610 (397.994, -103.8707) -> (397.8699, -103.8897)
  line L611 (397.8699, -103.8897) -> (397.7421, -103.8962)
  line L612 (397.7421, -103.8962) -> (397.6143, -103.8898)
  line L613 (397.6143, -103.8898) -> (397.4902, -103.8709)
  line L614 (397.4902, -103.8709) -> (397.3705, -103.8401)
  line L615 (397.3705, -103.8401) -> (397.2556, -103.7981)
  line L616 (397.2556, -103.7981) -> (397.1464, -103.7455)
  line L617 (397.1464, -103.7455) -> (397.0433, -103.6829)
  line L618 (397.0433, -103.6829) -> (396.947, -103.6109)
  line L619 (396.947, -103.6109) -> (396.8583, -103.5303)
  line L620 (396.8583, -103.5303) -> (396.7776, -103.4415)
  line L621 (396.7776, -103.4415) -> (396.7056, -103.3453)
  line L622 (396.7056, -103.3453) -> (396.643, -103.2423)
  line L623 (396.643, -103.2423) -> (396.5903, -103.133)
  line L624 (396.5903, -103.133) -> (396.5482, -103.0181)
  line L625 (396.5482, -103.0181) -> (396.5174, -102.8983)
  line L626 (396.5174, -102.8983) -> (396.4984, -102.7742)
  line L627 (396.4984, -102.7742) -> (396.4919, -102.6464)
  line L628 (396.4919, -102.6464) -> (396.4983, -102.5186)
  line L629 (396.4983, -102.5186) -> (396.5172, -102.3945)
  line L630 (396.5172, -102.3945) -> (396.548, -102.2747)
  line L631 (396.548, -102.2747) -> (396.59, -102.1599)
  line L632 (396.59, -102.1599) -> (396.6426, -102.0506)
  line L633 (396.6426, -102.0506) -> (396.7052, -101.9475)
  line L634 (396.7052, -101.9475) -> (396.7771, -101.8513)
  line L635 (396.7771, -101.8513) -> (396.8578, -101.7625)
  line L636 (396.8578, -101.7625) -> (396.9465, -101.6818)
  line L637 (396.9465, -101.6818) -> (397.0427, -101.6098)
  line L638 (397.0427, -101.6098) -> (397.1458, -101.5472)
  line L639 (397.1458, -101.5472) -> (397.255, -101.4945)
  line L640 (397.255, -101.4945) -> (397.3699, -101.4525)
  line L641 (397.3699, -101.4525) -> (397.4897, -101.4216)
  line L642 (397.4897, -101.4216) -> (397.6138, -101.4027)
  line L643 (397.6138, -101.4027) -> (397.7416, -101.3962)
  line L644 (354.6329, -89.6425) -> (354.6329, -86.2414)
  arc A0 (354.6329, -86.2414) -> (352.7945, -84.4029) centre (353.7137, -85.3221) ccw
  line L645 (352.7945, -84.4029) -> (327.4791, -84.4029)
  arc A1 (327.4791, -84.4029) -> (325.6406, -86.2414) centre (326.5598, -85.3221) ccw
  line L646 (325.6406, -86.2414) -> (325.6406, -89.6425)
  line L647 (325.6406, -89.6425) -> (325.6406, -95.6442)
  line L648 (325.6406, -95.6442) -> (325.6406, -99.077)
  arc A2 (325.6406, -99.077) -> (327.4791, -100.9155) centre (326.5598, -99.9963) ccw
  line L649 (327.4791, -100.9155) -> (352.7945, -100.9155)
  arc A3 (352.7945, -100.9155) -> (354.6329, -99.077) centre (353.7137, -99.9963) ccw
  line L650 (354.6329, -99.077) -> (354.6329, -95.6442)
  line L651 (354.6329, -95.6442) -> (354.6329, -89.6425)
  line L652 (354.6329, -9.6515) -> (354.6329, -6.2187)
  arc A4 (354.6329, -6.2187) -> (352.7945, -4.3802) centre (353.7137, -5.2994) ccw
  line L653 (352.7945, -4.3802) -> (327.4791, -4.3802)
  arc A5 (327.4791, -4.3802) -> (325.6406, -6.2187) centre (326.5598, -5.2994) ccw
  line L654 (325.6406, -6.2187) -> (325.6406, -9.6515)
  line L655 (325.6406, -9.6515) -> (325.6406, -15.6532)
  line L656 (325.6406, -15.6532) -> (325.6406, -19.0543)
  arc A6 (325.6406, -19.0543) -> (327.4791, -20.8928) centre (326.5598, -19.9736) ccw
  line L657 (327.4791, -20.8928) -> (352.7945, -20.8928)
  arc A7 (352.7945, -20.8928) -> (354.6329, -19.0543) centre (353.7137, -19.9736) ccw
  line L658 (354.6329, -19.0543) -> (354.6329, -15.6532)
  line L659 (354.6329, -15.6532) -> (354.6329, -9.6515)
  line L660 (411.2537, -15.6532) -> (411.2537, -19.0543)
  arc A8 (409.4152, -20.8928) -> (411.2537, -19.0543) centre (410.3344, -19.9736) ccw
  line L661 (409.4152, -20.8928) -> (384.0681, -20.8928)
  arc A9 (382.2296, -19.0543) -> (384.0681, -20.8928) centre (383.1488, -19.9736) ccw
  line L662 (382.2296, -19.0543) -> (382.2296, -15.6532)
  line L663 (382.2296, -15.6532) -> (382.2296, -9.6515)
  line L664 (382.2296, -9.6515) -> (382.2296, -6.2187)
  arc A10 (384.0681, -4.3802) -> (382.2296, -6.2187) centre (383.1488, -5.2994) ccw
  line L665 (384.0681, -4.3802) -> (409.4152, -4.3802)
  arc A11 (411.2537, -6.2187) -> (409.4152, -4.3802) centre (410.3344, -5.2994) ccw
  line L666 (411.2537, -6.2187) -> (411.2537, -9.6515)
  line L667 (411.2537, -9.6515) -> (411.2537, -15.6532)
  line L668 (405.4313, -48.7797) -> (405.5855, -48.7874)
  line L669 (405.5855, -48.7874) -> (405.7353, -48.8103)
  line L670 (405.7353, -48.8103) -> (405.8799, -48.8474)
  line L671 (405.8799, -48.8474) -> (406.0185, -48.8981)
  line L672 (406.0185, -48.8981) -> (406.1503, -48.9616)
  line L673 (406.1503, -48.9616) -> (406.2747, -49.0371)
  line L674 (406.2747, -49.0371) -> (406.3908, -49.124)
  line L675 (406.3908, -49.124) -> (406.498, -49.2213)
  line L676 (406.498, -49.2213) -> (406.5953, -49.3284)
  line L677 (406.5953, -49.3284) -> (406.6822, -49.4445)
  line L678 (406.6822, -49.4445) -> (406.7577, -49.5689)
  line L679 (406.7577, -49.5689) -> (406.8213, -49.7007)
  line L680 (406.8213, -49.7007) -> (406.872, -49.8393)
  line L681 (406.872, -49.8393) -> (406.9092, -49.9839)
  line L682 (406.9092, -49.9839) -> (406.9321, -50.1336)
  line L683 (406.9321, -50.1336) -> (406.9399, -50.2879)
  line L684 (406.9399, -50.2879) -> (406.9322, -50.4421)
  line L685 (406.9322, -50.4421) -> (406.9093, -50.5918)
  line L686 (406.9093, -50.5918) -> (406.8722, -50.7364)
  line L687 (406.8722, -50.7364) -> (406.8215, -50.875)
  line L688 (406.8215, -50.875) -> (406.758, -51.0068)
  line L689 (406.758, -51.0068) -> (406.6825, -51.1312)
  line L690 (406.6825, -51.1312) -> (406.5957, -51.2473)
  line L691 (406.5957, -51.2473) -> (406.4984, -51.3545)
  line L692 (406.4984, -51.3545) -> (406.3913, -51.4518)
  line L693 (406.3913, -51.4518) -> (406.2752, -51.5387)
  line L694 (406.2752, -51.5387) -> (406.1508, -51.6142)
  line L695 (406.1508, -51.6142) -> (406.019, -51.6778)
  line L696 (406.019, -51.6778) -> (405.8804, -51.7285)
  line L697 (405.8804, -51.7285) -> (405.7359, -51.7657)
  line L698 (405.7359, -51.7657) -> (405.5861, -51.7886)
  line L699 (405.5861, -51.7886) -> (405.4319, -51.7964)
  line L700 (405.4319, -51.7964) -> (405.2777, -51.7886)
  line L701 (405.2777, -51.7886) -> (405.1279, -51.7658)
  line L702 (405.1279, -51.7658) -> (404.9833, -51.7287)
  line L703 (404.9833, -51.7287) -> (404.8447, -51.678)
  line L704 (404.8447, -51.678) -> (404.7129, -51.6145)
  line L705 (404.7129, -51.6145) -> (404.5885, -51.539)
  line L706 (404.5885, -51.539) -> (404.4724, -51.4522)
  line L707 (404.4724, -51.4522) -> (404.3652, -51.3549)
  line L708 (404.3652, -51.3549) -> (404.2678, -51.2478)
  line L709 (404.2678, -51.2478) -> (404.181, -51.1317)
  line L710 (404.181, -51.1317) -> (404.1054, -51.0073)
  line L711 (404.1054, -51.0073) -> (404.0418, -50.8755)
  line L712 (404.0418, -50.8755) -> (403.9911, -50.7369)
  line L713 (403.9911, -50.7369) -> (403.9539, -50.5924)
  line L714 (403.9539, -50.5924) -> (403.931, -50.4426)
  line L715 (403.931, -50.4426) -> (403.9232, -50.2884)
  line L716 (403.9232, -50.2884) -> (403.9309, -50.1342)
  line L717 (403.9309, -50.1342) -> (403.9538, -49.9844)
  line L718 (403.9538, -49.9844) -> (403.9909, -49.8398)
  line L719 (403.9909, -49.8398) -> (404.0416, -49.7012)
  line L720 (404.0416, -49.7012) -> (404.1051, -49.5694)
  line L721 (404.1051, -49.5694) -> (404.1806, -49.445)
  line L722 (404.1806, -49.445) -> (404.2674, -49.3288)
  line L723 (404.2674, -49.3288) -> (404.3647, -49.2217)
  line L724 (404.3647, -49.2217) -> (404.4718, -49.1243)
  line L725 (404.4718, -49.1243) -> (404.5879, -49.0375)
  line L726 (404.5879, -49.0375) -> (404.7123, -48.9619)
  line L727 (404.7123, -48.9619) -> (404.8441, -48.8983)
  line L728 (404.8441, -48.8983) -> (404.9827, -48.8476)
  line L729 (404.9827, -48.8476) -> (405.1273, -48.8104)
  line L730 (405.1273, -48.8104) -> (405.277, -48.7875)
  line L731 (405.277, -48.7875) -> (405.4313, -48.7797)
  line L732 (331.4307, -48.7797) -> (331.5849, -48.7874)
  line L733 (331.5849, -48.7874) -> (331.7347, -48.8103)
  line L734 (331.7347, -48.8103) -> (331.8793, -48.8474)
  line L735 (331.8793, -48.8474) -> (332.0179, -48.8981)
  line L736 (332.0179, -48.8981) -> (332.1497, -48.9616)
  line L737 (332.1497, -48.9616) -> (332.2741, -49.0371)
  line L738 (332.2741, -49.0371) -> (332.3903, -49.124)
  line L739 (332.3903, -49.124) -> (332.4974, -49.2213)
  line L740 (332.4974, -49.2213) -> (332.5947, -49.3284)
  line L741 (332.5947, -49.3284) -> (332.6816, -49.4445)
  line L742 (332.6816, -49.4445) -> (332.7572, -49.5689)
  line L743 (332.7572, -49.5689) -> (332.8207, -49.7007)
  line L744 (332.8207, -49.7007) -> (332.8714, -49.8393)
  line L745 (332.8714, -49.8393) -> (332.9086, -49.9839)
  line L746 (332.9086, -49.9839) -> (332.9315, -50.1336)
  line L747 (332.9315, -50.1336) -> (332.9393, -50.2879)
  line L748 (332.9393, -50.2879) -> (332.9316, -50.4421)
  line L749 (332.9316, -50.4421) -> (332.9088, -50.5918)
  line L750 (332.9088, -50.5918) -> (332.8716, -50.7364)
  line L751 (332.8716, -50.7364) -> (332.8209, -50.875)
  line L752 (332.8209, -50.875) -> (332.7574, -51.0068)
  line L753 (332.7574, -51.0068) -> (332.6819, -51.1312)
  line L754 (332.6819, -51.1312) -> (332.5951, -51.2473)
  line L755 (332.5951, -51.2473) -> (332.4978, -51.3545)
  line L756 (332.4978, -51.3545) -> (332.3907, -51.4518)
  line L757 (332.3907, -51.4518) -> (332.2746, -51.5387)
  line L758 (332.2746, -51.5387) -> (332.1503, -51.6142)
  line L759 (332.1503, -51.6142) -> (332.0184, -51.6778)
  line L760 (332.0184, -51.6778) -> (331.8798, -51.7285)
  line L761 (331.8798, -51.7285) -> (331.7353, -51.7657)
  line L762 (331.7353, -51.7657) -> (331.5855, -51.7886)
  line L763 (331.5855, -51.7886) -> (331.4313, -51.7964)
  line L764 (331.4313, -51.7964) -> (331.2771, -51.7886)
  line L765 (331.2771, -51.7886) -> (331.1273, -51.7658)
  line L766 (331.1273, -51.7658) -> (330.9828, -51.7287)
  line L767 (330.9828, -51.7287) -> (330.8442, -51.678)
  line L768 (330.8442, -51.678) -> (330.7123, -51.6145)
  line L769 (330.7123, -51.6145) -> (330.5879, -51.539)
  line L770 (330.5879, -51.539) -> (330.4718, -51.4522)
  line L771 (330.4718, -51.4522) -> (330.3646, -51.3549)
  line L772 (330.3646, -51.3549) -> (330.2673, -51.2478)
  line L773 (330.2673, -51.2478) -> (330.1804, -51.1317)
  line L774 (330.1804, -51.1317) -> (330.1048, -51.0073)
  line L775 (330.1048, -51.0073) -> (330.0413, -50.8755)
  line L776 (330.0413, -50.8755) -> (329.9905, -50.7369)
  line L777 (329.9905, -50.7369) -> (329.9533, -50.5924)
  line L778 (329.9533, -50.5924) -> (329.9304, -50.4426)
  line L779 (329.9304, -50.4426) -> (329.9226, -50.2884)
  line L780 (329.9226, -50.2884) -> (329.9304, -50.1342)
  line L781 (329.9304, -50.1342) -> (329.9532, -49.9844)
  line L782 (329.9532, -49.9844) -> (329.9903, -49.8398)
  line L783 (329.9903, -49.8398) -> (330.041, -49.7012)
  line L784 (330.041, -49.7012) -> (330.1045, -49.5694)
  line L785 (330.1045, -49.5694) -> (330.18, -49.445)
  line L786 (330.18, -49.445) -> (330.2668, -49.3288)
  line L787 (330.2668, -49.3288) -> (330.3642, -49.2217)
  line L788 (330.3642, -49.2217) -> (330.4713, -49.1243)
  line L789 (330.4713, -49.1243) -> (330.5874, -49.0375)
  line L790 (330.5874, -49.0375) -> (330.7117, -48.9619)
  line L791 (330.7117, -48.9619) -> (330.8436, -48.8983)
  line L792 (330.8436, -48.8983) -> (330.9821, -48.8476)
  line L793 (330.9821, -48.8476) -> (331.1267, -48.8104)
  line L794 (331.1267, -48.8104) -> (331.2765, -48.7875)
  line L795 (331.2765, -48.7875) -> (331.4307, -48.7797)
  line L796 (411.2537, -89.6425) -> (411.2537, -86.2414)
  arc A12 (411.2537, -86.2414) -> (409.4152, -84.4029) centre (410.3344, -85.3221) ccw
  line L797 (409.4152, -84.4029) -> (384.0681, -84.4029)
  arc A13 (384.0681, -84.4029) -> (382.2296, -86.2414) centre (383.1488, -85.3221) ccw
  line L798 (382.2296, -86.2414) -> (382.2296, -89.6425)
  line L799 (382.2296, -89.6425) -> (382.2296, -95.6442)
  line L800 (382.2296, -95.6442) -> (382.2296, -99.077)
  arc A14 (382.2296, -99.077) -> (384.0681, -100.9155) centre (383.1488, -99.9963) ccw
  line L801 (384.0681, -100.9155) -> (409.4152, -100.9155)
  arc A15 (409.4152, -100.9155) -> (411.2537, -99.077) centre (410.3344, -99.9963) ccw
  line L802 (411.2537, -99.077) -> (411.2537, -95.6442)
  line L803 (411.2537, -95.6442) -> (411.2537, -89.6425)
  arc A16 (319.3354, -74.7443) -> (313.2354, -80.8443) centre (319.3354, -80.8443) ccw
  arc A17 (313.2354, -80.8443) -> (319.3354, -86.9443) centre (319.3354, -80.8443) ccw
  arc A18 (319.3354, -86.9443) -> (325.4354, -80.8443) centre (319.3354, -80.8443) ccw
  arc A19 (325.4354, -80.8443) -> (319.3354, -74.7443) centre (319.3354, -80.8443) ccw
  arc A20 (319.9977, -71.7474) -> (319.9917, -5.7474) centre (214.6703, -38.757) ccw
  line L804 (319.9917, -5.7474) -> (319.9856, 0.3592)
  line L805 (319.9856, 0.3592) -> (319.9998, 0.5635)
  line L806 (319.9998, 0.5635) -> (320.0414, 0.7617)
  line L807 (320.0414, 0.7617) -> (320.1091, 0.953)
  line L808 (320.1091, 0.953) -> (320.2015, 1.1362)
  line L809 (320.2015, 1.1362) -> (320.3174, 1.3105)
  line L810 (320.3174, 1.3105) -> (320.4552, 1.4748)
  line L811 (320.4552, 1.4748) -> (320.6136, 1.6281)
  line L812 (320.6136, 1.6281) -> (320.7914, 1.7694)
  line L813 (320.7914, 1.7694) -> (320.987, 1.8979)
  line L814 (320.987, 1.8979) -> (321.1992, 2.0124)
  line L815 (321.1992, 2.0124) -> (321.4266, 2.112)
  line L816 (321.4266, 2.112) -> (321.6679, 2.1957)
  line L817 (321.6679, 2.1957) -> (321.9215, 2.2625)
  line L818 (321.9215, 2.2625) -> (322.1863, 2.3115)
  line L819 (322.1863, 2.3115) -> (322.4608, 2.3416)
  line L820 (322.4608, 2.3416) -> (322.7436, 2.3519)
  line L821 (322.7436, 2.3519) -> (347.685, 2.3503)
  line L822 (347.685, 2.3503) -> (348.2935, 2.114)
  line L823 (348.2935, 2.114) -> (348.9059, 1.8851)
  line L824 (348.9059, 1.8851) -> (349.5221, 1.6638)
  line L825 (349.5221, 1.6638) -> (350.1418, 1.4499)
  line L826 (350.1418, 1.4499) -> (350.7651, 1.2436)
  line L827 (350.7651, 1.2436) -> (351.3916, 1.0448)
  line L828 (351.3916, 1.0448) -> (352.0214, 0.8535)
  line L829 (352.0214, 0.8535) -> (352.6544, 0.6697)
  line L830 (352.6544, 0.6697) -> (353.2903, 0.4934)
  line L831 (353.2903, 0.4934) -> (353.929, 0.3246)
  line L832 (353.929, 0.3246) -> (354.5705, 0.1633)
  line L833 (354.5705, 0.1633) -> (355.2146, 0.0095)
  line L834 (355.2146, 0.0095) -> (355.8612, -0.1368)
  line L835 (355.8612, -0.1368) -> (356.5101, -0.2756)
  line L836 (356.5101, -0.2756) -> (357.1613, -0.4069)
  line L837 (357.1613, -0.4069) -> (357.8146, -0.5306)
  line L838 (357.8146, -0.5306) -> (358.4699, -0.6469)
  line L839 (358.4699, -0.6469) -> (359.127, -0.7557)
  line L840 (359.127, -0.7557) -> (359.7859, -0.8569)
  line L841 (359.7859, -0.8569) -> (360.4464, -0.9507)
  line L842 (360.4464, -0.9507) -> (361.1084, -1.0369)
  line L843 (361.1084, -1.0369) -> (361.7717, -1.1157)